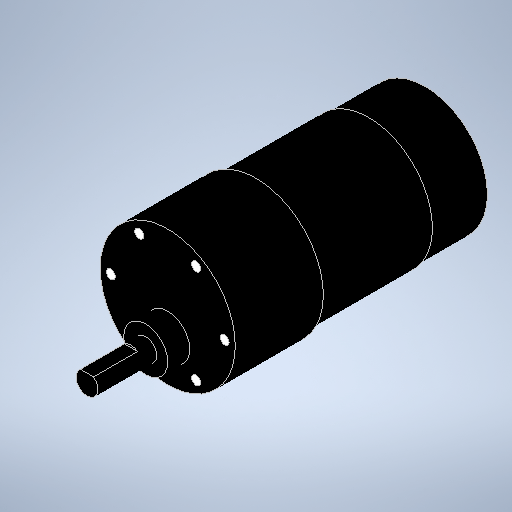
# Autodesk Inventor part: Metal Gearmotor
Saved by Autodesk Inventor 2026.2 (Build 302298010, 298A)
## iProperties
Created: 2026-05-06
Part Number: Metal Gearmotor
Material: 一般
Document SubType Name: Modeling
Designer: Yagis
Density: 1 g/cm^3
Appearance: 既定
Author: Yagis
Autodesk Inventor part; units mm, degrees
ref_plane "YZ Plane" through (0, 0, 0) normal (1, 0, 0) x (0, 1, 0)
ref_plane "XZ Plane" through (0, 0, 0) normal (0, 1, 0) x (-1, 0, 0)
ref_plane "XY Plane" through (0, 0, 0) normal (0, 0, 1) x (1, 0, 0)
sketch "スケッチ1" plane through (0, 0, 0) normal (0, 0, 1) x (1, 0, 0)
  circle A0 centre (0, 0) radius 18.4
  constraints: 1 centre point, 1 coincident
extrude "押し出し1" add sketch "スケッチ1" along normal blind 24
sketch "スケッチ2" plane through (0, 0, 0) normal (0, 0, -1) x (-1, 0, 0)
  circle A0 centre (0, 0) radius 17.4
  dimension "d3" = 34.8
  constraints: 1 centre point, 1 coincident
  measures "d3" diameter of A0
extrude "押し出し2" add sketch "スケッチ2" along normal blind 30.7
sketch "スケッチ3" plane through (0, 0, -30.7) normal (0, 0, -1) x (-1, 0, 0)
  circle A0 centre (0, 0) radius 17
  dimension "d6" = 34
  constraints: 1 centre point, 1 coincident
  measures "d6" diameter of A0
extrude "押し出し3" add sketch "スケッチ3" along normal blind 15.4
sketch "スケッチ4" plane through (0, 0, 24) normal (0, 0, 1) x (1, 0, 0)
  circle A0 centre (0, -7) radius 6
  circle A1 centre (0, -7) radius 3
  point P0 (0, 0)
  point P1 (-15.5, 0)
  point P2 (0, 0)
  point P3 (-7.75, -13.4234)
  point P4 (7.75, -13.4234)
  point P5 (15.5, 0)
  point P6 (7.75, 13.4234)
  point P7 (-7.75, 13.4234)
  dimension "d11" = 360
  dimension "d13" = 15.5
  dimension "d14" = 7
  dimension "d15" = 12
  dimension "d16" = 6
  constraints: 2 centre point, 2 coincident, 7 other
  measures "d13" distance of point (-15.5, 0) point (0, 0)
  measures "d14" distance of point (0, 0) A0.centre
  measures "d15" diameter of A0
  measures "d16" diameter of A1
extrude "押し出し4" add sketch "スケッチ4" along normal blind 6
extrude "押し出し5" add sketch "スケッチ4" along normal blind 22 contours A1
sketch "スケッチ5" plane through (0, -7, 46) normal (0, 0, 1) x (1, 0, 0)
  circle A0 centre (0, 0) radius 3
  line L0 (0, 2.4) -> (1.8, 2.4)
  line L1 (0, 2.4) -> (-1.8, 2.4)
  point P0 (0, 7)
  dimension "d21" = 6
  dimension "d22" = 2.4
  constraints: 4 end point, 2 horizontal, 2 point on circle, 1 centre point
  measures "d21" diameter of A0
  measures "d22" distance of A0.centre L0.start
extrude "押し出し6" cut sketch "スケッチ5" against normal blind 12 contours L0 L1 A0 picked at (-1.016, 2.5094)
sketch "スケッチ6" plane through (0, 0, 24) normal (0, 0, 1) x (1, 0, 0)
  point P0 (0, 0)
  point P1 (-15.5, 0)
  point P2 (-7.75, -13.4234)
  point P3 (7.75, -13.4234)
  point P4 (15.5, 0)
  point P5 (7.75, 13.4234)
  point P6 (-7.75, 13.4234)
  dimension "d25" = 15.5
  dimension "d28" = 360
  constraints: 7 other
  measures "d25" distance of point (-15.5, 0) point (0, 0)
hole "穴1" at (7.75, 13.4234, 24) at (-7.75, 13.4234, 24) at (-15.5, 0, 24) at (-7.75, -13.4234, 24) at (7.75, -13.4234, 24) at (15.5, 0, 24) direction (0, 0, -1) diameter 2.459 depth 8.8 tip angle 118 thread size "M3x0.5" class "6H" standard "ISO Metric profile"
